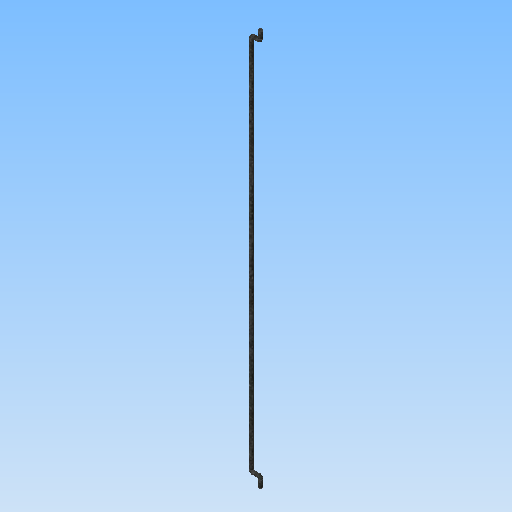
# Autodesk Inventor part: Selection_Wire
Saved by Autodesk Inventor 2018.1 (Build 221171000, 171)
## iProperties
Created: 2019-02-22
Part Number: Selection_Wire
Material: Steel
Document SubType Name: Modeling
Designer: James
Density: 7.85 g/cm^3
Appearance: Plate
Mass: 5.58048 g
Surface Area: 14.2806 cm^2
Volume: 0.71089 cm^3
Author: James
Autodesk Inventor part; units mm, degrees
ref_plane "YZ Plane" through (0, 0, 0) normal (1, 0, 0) x (0, 1, 0)
ref_plane "XZ Plane" through (0, 0, 0) normal (0, 1, 0) x (-1, 0, 0)
ref_plane "XY Plane" through (0, 0, 0) normal (0, 0, 1) x (1, 0, 0)
sketch "Sketch2" plane through (0, 0, 0) normal (0, 1, 0) x (-1, 0, 0)
  circle A0 centre (0, 0) radius 1
  dimension "d0" = 2
  constraints: 1 centre point, 1 coincident
  measures "d0" diameter of A0
sketch "Sketch3" plane through (0, 0, 0) normal (0, 0, 1) x (1, 0, 0)
  line L0 (0, 0) -> (0, -4)
  line L1 (-1, -5) -> (-4, -5)
  line L2 (-5, -6) -> (-5, -212)
  line L3 (-4, -213) -> (-1, -213)
  line L4 (0, -214) -> (0, -218)
  arc A0 (-1, -5) -> (0, -4) centre (-1, -4) ccw
  arc A1 (-4, -5) -> (-5, -6) centre (-4, -6) ccw
  arc A2 (-5, -212) -> (-4, -213) centre (-4, -212) ccw
  arc A3 (0, -214) -> (-1, -213) centre (-1, -214) ccw
  point P0 (0, -5)
  point P1 (-5, -5)
  point P2 (-5, -213)
  point P3 (0, -213)
  dimension "d1" = 5
  dimension "d2" = 5
  dimension "d3" = 5
  dimension "d4" = 208
  dimension "d7" = 1
  dimension "d8" = 1
  dimension "d9" = 1
  constraints: 10 end point, 10 point on line, 8 point on circle, 8 tangent, 4 centre point, 3 perpendicular, 1 equal radius, 1 vertical
  measures "d1" distance of L0.start point (0, -5)
  measures "d2" distance of point (0, -213) L4.end
  measures "d3" distance of point (0, -5) point (-5, -5)
  measures "d4" distance of point (-5, -5) point (-5, -213)
  measures "d7" radius of A0
  measures "d8" radius of A1
  measures "d9" radius of A3
sweep "Sweep1" add profiles "Sketch2" path "Sketch3"
equation "\"d2\" = d1"
body "Solid1"
